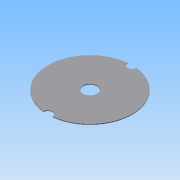
# Autodesk Inventor part: 零件2
Saved by Autodesk Inventor 2015 (Build 190159000, 159)
## iProperties
Created: 2018-04-17
Part Number: 零件2
Material: 一般
Document SubType Name: Modeling
Designer: 王博聖
Density: 1 g/cm^3
Appearance: 預設
Author: 王博聖
Autodesk Inventor part; units mm, degrees
ref_plane "YZ Plane" through (0, 0, 0) normal (1, 0, 0) x (0, 1, 0)
ref_plane "XZ Plane" through (0, 0, 0) normal (0, 1, 0) x (-1, 0, 0)
ref_plane "XY Plane" through (0, 0, 0) normal (0, 0, 1) x (1, 0, 0)
sketch "草圖1" plane through (0, 0, 0) normal (0, 0, 1) x (1, 0, 0)
  circle A0 centre (0, 0) radius 10
  dimension "d0" = 20
  constraints: 1 centre point, 1 coincident
  measures "d0" diameter of A0
extrude "擠出1" add sketch "草圖1" along normal blind 17
sketch "草圖2" plane through (0, 0, 0) normal (0, 0, -1) x (-1, 0, 0)
  circle A0 centre (0, 0) radius 10 projected
  circle A1 centre (0, 0) radius 60
  line L0 (0, 0) -> (0, 60)
  circle A2 centre (0, 60) radius 6.5
  dimension "d3" = 120
  dimension "d4" = 13
  constraints: 2 coincident, 2 end point, 1 centre point, 1 vertical, 1 vertical alignment, 2 other
  measures "d4" diameter of A2
extrude "擠出2" add sketch "草圖2" along normal blind 1 contours A0 | A2 A1 | A2 A1 L0 | L0 A1 A2 picked at (-11.4207, 38.8636)
extrude "擠出3" cut sketch "草圖2" along normal blind 1 contours A2 A1 L0 | L0 A1 A2 | A1 A2 picked at (1.4483, 62.0284)
pattern_circular "環形陣列1" count 2 over 360 about axis through (0, 0, 0) along (0, 0, -1) of "擠出3"
sketch "草圖3" plane through (0, 0, 17) normal (0, 0, 1) x (1, 0, 0)
  circle A0 centre (0, 0) radius 10 projected
extrude "擠出4" cut sketch "草圖3" against normal blind 65
